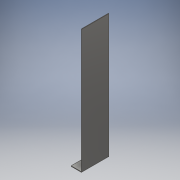
# Autodesk Inventor part: Feder
Saved by Autodesk Inventor 2019 (Build 230136000, 136)
## iProperties
Created: 2020-04-12
Part Number: Feder
Material: Stainless Steel
Document SubType Name: Modeling
Designer: Erle
Density: 8 g/cm^3
Appearance: Semi-Polished
Mass: 0.3968 g
Surface Area: 5.08203 cm^2
Volume: 0.0496 cm^3
Author: Erle
Autodesk Inventor part; units mm, degrees
ref_plane "YZ Plane" through (0, 0, 0) normal (1, 0, 0) x (0, 1, 0)
ref_plane "XZ Plane" through (0, 0, 0) normal (0, 1, 0) x (-1, 0, 0)
ref_plane "XY Plane" through (0, 0, 0) normal (0, 0, 1) x (1, 0, 0)
sketch "Sketch1" plane through (0, 0, 0) normal (0, 0, 1) x (1, 0, 0)
  line L0 (-4, 0) -> (0, 0)
  line L1 (0, 0) -> (0, 46)
  line L2 (0, 46) -> (-0.2, 46)
  line L3 (-0.2, 46) -> (-0.2, 0.2)
  line L4 (-0.2, 0.2) -> (-4, 0.2)
  line L5 (-4, 0.2) -> (-4, 0)
  dimension "d0" = 0.2
  dimension "d1" = 0.2
  dimension "d2" = 46
  dimension "d3" = 4
  constraints: 12 end point, 5 perpendicular, 1 horizontal
  measures "d0" distance of L1.end L2.end
  measures "d1" distance of L4.end L0.start
  measures "d2" distance of L0.end L1.end
  measures "d3" distance of L0.start L0.end
extrude "Extrusion1" add sketch "Sketch1" along normal blind 10
fillet "Fillet1" radius 0.2 2 edges at (0, 0, 5) (-0.2, 0.2, 5)
body "Solid1"
